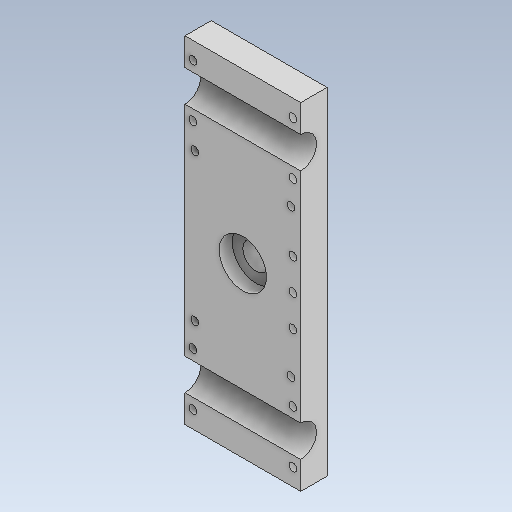
# Autodesk Inventor part: YClamp
Saved by Autodesk Inventor 2020 (Build 240168000, 168)
## iProperties
Created: 2020-03-18
Part Number: YClamp
Material: Generic
Document SubType Name: Modeling
Designer: DasNick
Density: 1 g/cm^3
Appearance: Default
Author: DasNick
Autodesk Inventor part; units mm, degrees
ref_plane "YZ Plane" through (0, 0, 0) normal (1, 0, 0) x (0, 1, 0)
ref_plane "XZ Plane" through (0, 0, 0) normal (0, 1, 0) x (-1, 0, 0)
ref_plane "XY Plane" through (0, 0, 0) normal (0, 0, 1) x (1, 0, 0)
sketch "Sketch1" plane through (0, 0, 0) normal (0, 0, 1) x (1, 0, 0)
  line L0 (-23.6094, 98.425) -> (-0.1834, 98.425) projected
  line L1 (-0.1834, 150.8125) -> (-0.1834, 98.425) projected
  line L2 (-23.6094, 150.8125) -> (-0.1834, 150.8125) projected
  line L3 (-23.6094, 150.8125) -> (-23.6094, 98.425) projected
  circle A0 centre (-18.8469, 140.4937) radius 2.3813 projected
  circle A1 centre (-18.8469, 108.7437) radius 2.3812 projected
  line L4 (-23.6094, -52.3875) -> (-0.1834, -52.3875) projected
  line L5 (-0.1834, 0) -> (-0.1834, -52.3875) projected
  line L6 (-23.6094, 0) -> (0, 0) projected
  line L7 (-23.6094, 0) -> (-23.6094, -52.3875) projected
  circle A2 centre (-18.8469, -10.3188) radius 2.3813 projected
  circle A3 centre (-18.8469, -42.0688) radius 2.3813 projected
  line L8 (22.8147, 98.425) -> (46.2406, 98.425) projected
  line L9 (46.2406, 150.8125) -> (46.2406, 98.425) projected
  line L10 (22.8147, 150.8125) -> (46.2406, 150.8125) projected
  line L11 (22.8147, 150.8125) -> (22.8147, 98.425) projected
  circle A4 centre (41.4781, 140.4938) radius 2.3813 projected
  circle A5 centre (41.4781, 108.7438) radius 2.3813 projected
  line L12 (22.8147, -52.3875) -> (46.2406, -52.3875) projected
  line L13 (46.2406, 0) -> (46.2406, -52.3875) projected
  line L14 (22.8147, 0) -> (46.2406, 0) projected
  line L15 (22.8147, 0) -> (22.8147, -52.3875) projected
  circle A6 centre (41.4781, -10.3187) radius 2.3813 projected
  circle A7 centre (41.4781, -42.0687) radius 2.3813 projected
  line L16 (22.8147, 150.8125) -> (-0.1834, 150.8125)
  line L17 (22.8147, -52.3875) -> (-0.1834, -52.3875)
  line L18 (46.2406, 0) -> (46.2406, 98.425)
  line L19 (-23.6094, 0) -> (-23.6094, 98.425)
  constraints: 8 end point, 2 perpendicular, 1 collinear, 1 parallel
extrude "Extrusion1" add sketch "Sketch1" along normal blind 15.875
sketch "Sketch2" plane through (-23.6094, -52.3875, 0) normal (-1, 0, 0) x (0, 0, 1)
  line L0 (15.875, 195.2625) -> (15.875, 190.5) projected
  line L1 (15.875, 163.5125) -> (15.875, 158.75) projected
  line L2 (15.875, 44.45) -> (15.875, 39.6875) projected
  line L3 (15.875, 190.5) -> (15.875, 163.5125) construction
  line L4 (15.875, 12.7) -> (0, 12.7) construction
  line L5 (15.875, 12.7) -> (15.875, 39.6875) construction
  line L6 (22.1465, 177.0062) -> (15.875, 177.0062)
  line L7 (15.875, 0) -> (15.875, 203.2) projected
  line L8 (24.8676, 26.1938) -> (15.875, 26.1938)
  line L9 (15.875, 203.2) -> (15.875, 0) projected
  circle A0 centre (15.875, 177.0062) radius 9.525
  circle A1 centre (15.875, 26.1938) radius 9.525
  point P0 (0, 52.3875)
  point P1 (15.875, 35.7188)
  point P2 (15.875, 16.6688)
  point P3 (15.875, 186.5312)
  point P4 (15.875, 167.4812)
  dimension "d2" = 19.05
  dimension "d3" = 19.05
  constraints: 8 end point, 2 centre point, 2 coincident, 2 point on line, 1 collinear, 1 parallel, 1 perpendicular, 4 other
  measures "d2" diameter of A0
  measures "d3" diameter of A1
extrude "Extrusion2" cut sketch "Sketch2" against normal blind 76.2 contours L7 A1 | A0 L7 picked at (15.1152, 19.9361) picked at (15.1152, 170.7485)
sketch "Sketch3" plane through (0, 0, 15.875) normal (0, 0, 1) x (1, 0, 0)
  circle A0 centre (41.4781, 108.7438) radius 2.3813 construction
  circle A1 centre (41.4781, -10.3187) radius 2.3813 construction
  line L0 (41.4781, 108.7438) -> (41.4781, -10.3187) construction
  circle A2 centre (41.4781, 49.2125) radius 2.3813 construction
  circle A3 centre (41.4781, 30.1625) radius 2.3813 construction
  circle A4 centre (41.4781, 68.2625) radius 2.3813 construction
  circle A5 centre (41.4781, 49.2125) radius 2.3813 construction
  circle A6 centre (41.4781, 68.2625) radius 2.3813
  circle A7 centre (41.4781, 49.2125) radius 2.3813
  circle A8 centre (41.4781, 30.1625) radius 2.3813
  point P0 (0, 0)
  dimension "d8" = 19.05
  dimension "d11" = 19.05
  constraints: 7 centre point, 3 coincident, 3 concentric, 3 vertical, 2 end point, 1 midpoint, 6 other
  measures "d8" distance of A2.centre A3.centre
  measures "d11" distance of A2.centre A4.centre
extrude "Extrusion3" cut sketch "Sketch3" against normal blind 76.2
sketch "Sketch4" plane through (0, 0, 15.875) normal (0, 0, 1) x (1, 0, 0)
  circle A0 centre (11.3156, 49.2125) radius 14.2875
  line L0 (-23.6094, 115.0937) -> (-23.6094, -16.6688) projected
  point P0 (0, 0)
  dimension "d16" = 34.925
  dimension "d17" = 28.575
  constraints: 1 centre point
  measures "d16" distance from line of L0 A0.centre
  measures "d17" diameter of A0
extrude "Extrusion4" cut sketch "Sketch4" against normal blind 7.9375
sketch "Sketch5" plane through (11.3156, 49.2125, 7.9375) normal (0, 0, 1) x (1, 0, 0)
  circle A0 centre (0, 0) radius 7.9375
  point P0 (-11.3156, -49.2125)
  dimension "d20" = 15.875
  constraints: 1 centre point
  measures "d20" diameter of A0
extrude "Extrusion5" cut sketch "Sketch5" against normal blind 7.9375
sketch "Sketch6" plane through (0, 0, 15.875) normal (0, 0, 1) x (1, 0, 0)
  line L0 (-23.6094, 100.0125) -> (46.2406, 100.0125) projected
  line L1 (46.2406, -1.5875) -> (-23.6094, -1.5875) projected
  circle A0 centre (11.3156, 49.2125) radius 37.465 projected
  circle A1 centre (40.3188, 93.6625) radius 2.3813
  line L2 (48.7806, 49.2125) -> (-26.1494, 49.2125) construction
  line L3 (11.3156, 100.0125) -> (11.3156, -1.5875) construction
  circle A2 centre (40.3188, 4.7625) radius 2.3813
  circle A3 centre (-17.6876, 93.6625) radius 2.3813
  circle A4 centre (-17.6876, 4.7625) radius 2.3813
  point P0 (0, 0)
  dimension "d23" = 4.7625
  dimension "d24" = 6.35
  constraints: 4 centre point, 4 end point, 3 symmetric about line, 2 midpoint, 2 point on circle, 1 horizontal, 3 other
  measures "d23" diameter of A1
  measures "d24" distance from line of L0 A1.centre
extrude "Extrusion6" cut sketch "Sketch6" against normal blind 19.05 contours A1 | A2 | A3 | A4
sketch "Sketch7" plane through (0, 0, 0) normal (0, 0, -1) x (-1, 0, 0)
  point P0 (0, 0)
body "Solid1"
